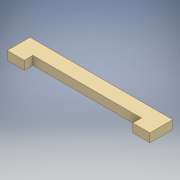
# Autodesk Inventor part: Celda pared cremallera
Saved by Autodesk Inventor 2018 (Build 220112000, 112)
## iProperties
Created: 2020-03-13
Part Number: Celda pared cremallera
Material: Genérico
Document SubType Name: Modeling
Designer: joser
Density: 1 g/cm^3
Appearance: Trigo
Author: joser
Autodesk Inventor part; units mm, degrees
ref_plane "YZ Plane" through (0, 0, 0) normal (1, 0, 0) x (0, 1, 0)
ref_plane "XZ Plane" through (0, 0, 0) normal (0, 1, 0) x (-1, 0, 0)
ref_plane "XY Plane" through (0, 0, 0) normal (0, 0, 1) x (1, 0, 0)
sketch "Boceto1" plane through (0, 0, 0) normal (0, 0, 1) x (1, 0, 0)
  line L0 (0, 8) -> (50, 8)
  line L1 (50, 8) -> (50, 0)
  line L2 (0, 0) -> (0, 8)
  line L3 (6, 0) -> (6, 3)
  line L4 (6, 3) -> (44, 3)
  line L5 (44, 3) -> (44, 0)
  line L6 (50, 0) -> (44, 0)
  line L7 (6, 0) -> (0, 0)
  dimension "d1" = 50
  dimension "d5" = 6
  dimension "d6" = 3
  dimension "d7" = 5
  dimension "d8" = 38
  constraints: 16 end point, 4 perpendicular, 3 parallel, 1 coincident, 1 collinear, 1 horizontal, 1 vertical
  measures "d1" distance between parallel lines of L1 L2
  measures "d5" distance between parallel lines of L2 L3
  measures "d6" distance between parallel lines of L7 L4
  measures "d7" distance between parallel lines of L0 L4
  measures "d8" distance between parallel lines of L5 L3
extrude "Extrusión1" add sketch "Boceto1" along normal blind 3
